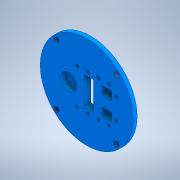
# Autodesk Inventor part: TE_01
Saved by Autodesk Inventor 2021 (Build 250183000, 183)
## iProperties
Created: 2022-04-22
Part Number: TE_01
Material: PETG
Document SubType Name: Modeling
Designer: Alcatraz
Density: 1.27 g/cm^3
Appearance: Genérico
Author: Alcatraz
Autodesk Inventor part; units mm, degrees
ref_plane "YZ Plane" through (0, 0, 0) normal (1, 0, 0) x (0, 1, 0)
ref_plane "XZ Plane" through (0, 0, 0) normal (0, 1, 0) x (-1, 0, 0)
ref_plane "XY Plane" through (0, 0, 0) normal (0, 0, 1) x (1, 0, 0)
sketch "Boceto1" plane through (0, 0, 0) normal (0, 0, 1) x (1, 0, 0)
  circle A0 centre (0, 0) radius 29
  dimension "Diametro" = 58
  constraints: 1 centre point, 1 coincident
  measures "Diametro" diameter of A0
extrude "Extrusión1" add sketch "Boceto1" along normal blind 5
sketch "Boceto2" plane through (0, 0, 5) normal (0, 0, 1) x (1, 0, 0)
  circle A0 centre (1, -13.5) radius 1
  arc A1 (11.666, -9.2) -> (12.466, -10) centre (12.466, -9.2) ccw
  line L0 (5.15, -10.5) -> (-1.85, -10.5)
  circle A2 centre (9, -13.5) radius 1
  line L1 (5.15, 10.5) -> (5.15, -10.5)
  line L2 (25, 16) -> (25, -16)
  line L3 (25, -16) -> (-25, -16)
  line L4 (-25, 16) -> (25, 16)
  line L5 (-25, -16) -> (25, 16) construction
  line L6 (25, -16) -> (-25, 16) construction
  arc A3 (18.866, -4.8) -> (18.066, -4) centre (18.066, -4.8) ccw
  line L7 (18.066, -4) -> (12.466, -4)
  line L8 (12.466, -10) -> (18.066, -10)
  line L9 (15.266, -4) -> (12.466, -4)
  line L10 (11.666, -4.8) -> (11.666, -9.2)
  line L11 (18.866, -9.2) -> (18.866, -4.8)
  arc A4 (12.466, -4) -> (11.666, -4.8) centre (12.466, -4.8) ccw
  line L12 (-1.85, -10.5) -> (-1.85, 0)
  circle A5 centre (-7, -13.5) radius 1
  line L13 (-25, -16) -> (-25, 16)
  line L14 (-1.85, 0) -> (-1.85, 10.5)
  circle A6 centre (-13.5, 0) radius 6
  circle A7 centre (1, 13.5) radius 1
  line L15 (-1.85, 10.5) -> (5.15, 10.5)
  circle A8 centre (-7, 13.5) radius 1
  arc A9 (18.066, -10) -> (18.866, -9.2) centre (18.066, -9.2) ccw
  circle A10 centre (22.5, -8) radius 1
  circle A11 centre (17, -13.5) radius 1
  circle A12 centre (9, 13.5) radius 1
  arc A13 (12.466, 10) -> (11.666, 9.2) centre (12.466, 9.2) ccw
  line L16 (11.666, 4.8) -> (11.666, 9.2)
  arc A14 (11.666, 4.8) -> (12.466, 4) centre (12.466, 4.8) ccw
  circle A15 centre (17, 13.5) radius 1
  line L17 (15.266, 4) -> (12.466, 4)
  line L18 (12.466, 10) -> (18.066, 10)
  arc A16 (18.866, 9.2) -> (18.066, 10) centre (18.066, 9.2) ccw
  line L19 (18.066, 4) -> (15.266, 4)
  line L20 (18.866, 9.2) -> (18.866, 4.8)
  arc A17 (18.066, 4) -> (18.866, 4.8) centre (18.066, 4.8) ccw
  circle A18 centre (22.5, 8) radius 1
  point P0 (0, 0)
  dimension "d3" = 50
  dimension "d4" = 32
  dimension "d5" = 12
  dimension "d6" = 11.65
  dimension "d7" = 10.5
  dimension "d8" = 7
  dimension "d9" = 21
  dimension "d10" = 2.8
  dimension "d11" = 4.4
  dimension "d12" = 5.6
  dimension "d13" = 4.4
  dimension "d14" = 0.8
  dimension "d15" = 0.8
  dimension "d16" = 0.8
  dimension "d17" = 0.8
  dimension "d18" = 0.8
  dimension "d19" = 0.8
  dimension "d20" = 2
  dimension "d21" = 2
  dimension "d22" = 2
  dimension "d23" = 2
  dimension "d24" = 2
  dimension "d25" = 2
  dimension "d26" = 2
  dimension "d27" = 2
  dimension "d28" = 2
  dimension "d29" = 2
  constraints: 42 end point, 19 centre point, 16 point on circle, 5 perpendicular, 4 tangent, 2 horizontal, 2 parallel, 2 point on line, 1 collinear, 1 vertical
  measures "d3" distance of L4.start L2.start
  measures "d4" distance of L3.end L4.start
  measures "d5" diameter of A6
  measures "d6" distance of A6.centre L14.start
  measures "d7" distance of L14.start L15.start
  measures "d8" distance of L15.start L15.end
  measures "d9" distance of L15.end L1.end
  measures "d10" distance of L17.start L17.end
  measures "d11" distance of L16.start L16.end
  measures "d12" distance of L18.start L18.end
  measures "d13" distance of L10.start L10.end
  measures "d14" radius of A4
  measures "d15" radius of A3
  measures "d16" radius of A9
  measures "d17" radius of A17
  measures "d18" radius of A16
  measures "d19" radius of A14
  measures "d20" diameter of A10
  measures "d21" diameter of A18
  measures "d22" diameter of A11
  measures "d23" diameter of A5
  measures "d24" diameter of A0
  measures "d25" diameter of A2
  measures "d26" diameter of A15
  measures "d27" diameter of A8
  measures "d28" diameter of A7
  measures "d29" diameter of A12
extrude "Extrusión2" cut sketch "Boceto2" against normal blind 3.2 contours L10 A4 L7 A3 L11 A9 L8 A1 | A6 | L18 A16 L20 A17 L19 L17 A14 L16 A13
extrude "Extrusión3" cut sketch "Boceto2" against normal blind 5 contours L0 L12 L14 L15 L1
sketch "Boceto3" plane through (0, 0, 5) normal (0, 0, 1) x (1, 0, 0)
  circle A0 centre (0, 0) radius 35
  circle A1 centre (0, 0) radius 29
  line L0 (0, 0) -> (22.6274, 22.6274)
  line L1 (0, 0) -> (32, 0) construction
  circle A2 centre (22.6274, 22.6274) radius 1.5
  circle A3 centre (-22.6274, 22.6274) radius 1.5
  circle A4 centre (-22.6274, -22.6274) radius 1.5
  circle A5 centre (22.6274, -22.6274) radius 1.5
  dimension "d34" = 70
  dimension "d35" = 58
  dimension "d40" = 32
  dimension "d41" = 45
  dimension "d42" = 3
  dimension "d45" = 360
  constraints: 6 centre point, 4 end point, 3 coincident, 1 equal length, 1 horizontal, 9 other
  measures "d34" diameter of A0
  measures "d35" diameter of A1
  measures "d40" distance of L0.start L0.end
  measures "d41" angle of L1 L0
  measures "d42" diameter of A2
extrude "Extrusión4" add sketch "Boceto3" against normal blind 3 contours A0 | A2 | A3 | A4 | A5
hole "Agujero1" at (22.6274, 22.6274, 5) at (-22.6274, 22.6274, 5) at (-22.6274, -22.6274, 5) at (22.6274, -22.6274, 5) direction (0, 0, -1) diameter 3.6881 depth 13 thread size "M4.5x0.75" class "6H" standard "ISO Metric profile"
hole "Agujero2" at (-7, -13.5, 5) at (1, -13.5, 5) at (9, -13.5, 5) at (17, -13.5, 5) at (22.5, -8, 5) at (22.5, 8, 5) at (17, 13.5, 5) at (9, 13.5, 5) at (1, 13.5, 5) at (-7, 13.5, 5) direction (0, 0, -1) diameter 2.013 depth 7.6 thread size "M2.5x0.45" class "6H" standard "ISO Metric profile"
equation "\"d35\" = Diametro"
